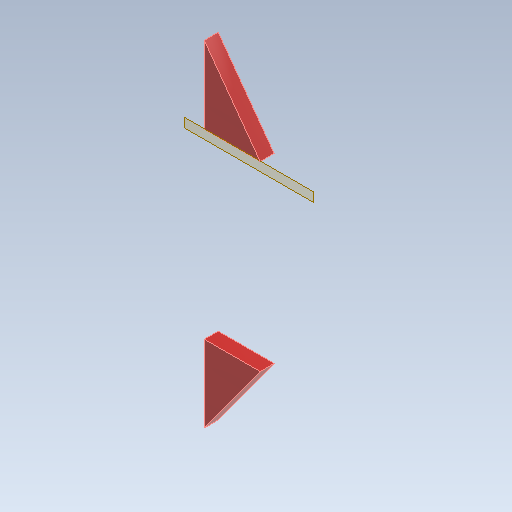
# Autodesk Inventor part: supportForFileHanger
Saved by Autodesk Inventor 2021 (Build 250183000, 183)
## iProperties
Created: 2020-07-03
Part Number: supportForFileHanger
Material: PET Plastic
Document SubType Name: Modeling
Designer: robst
Density: 1.541 g/cm^3
Appearance: Orange-Red
Author: robst
Autodesk Inventor part; units mm, degrees
ref_plane "YZ Plane" through (0, 0, 0) normal (1, 0, 0) x (0, 1, 0)
ref_plane "XZ Plane" through (0, 0, 0) normal (0, 1, 0) x (-1, 0, 0)
ref_plane "XY Plane" through (0, 0, 0) normal (0, 0, 1) x (1, 0, 0)
ref_plane "Work Plane1" through (0, 0, 0) normal (0, 0, 1) x (1, 0, 0)
sketch "Sketch1" plane through (0, 0, 0) normal (0, 0, 1) x (1, 0, 0)
  line L0 (53.34, 1.905) -> (0, 1.905)
  line L1 (0, -80.645) -> (53.34, -80.645)
  line L2 (6.35, 36.83) -> (0, 36.83)
  line L3 (6.35, -115.57) -> (0, -115.57)
  line L4 (0, 1.905) -> (8.89, 1.905)
  line L5 (0, 1.905) -> (8.89, 1.905)
  line L6 (0, 1.905) -> (8.89, 1.905)
  line L7 (6.35, -80.645) -> (6.35, -115.57)
  line L8 (6.35, -115.57) -> (31.75, -80.645)
  line L9 (31.75, -80.645) -> (6.35, -80.645)
  line L10 (6.35, 36.83) -> (31.75, 1.905)
  line L11 (31.75, 1.905) -> (6.35, 1.905)
  line L12 (6.35, 1.905) -> (6.35, 36.83)
  point P0 (0, 0)
  point P1 (6.35, 1.905)
extrude "Extrusion1" add sketch "Sketch1" against normal blind 6.35
body "Solid1"
